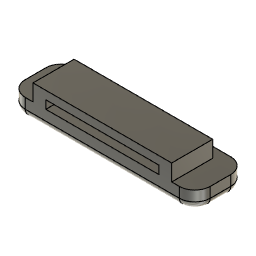
Keyboard_tray_end_stop_v5 (Autodesk Fusion 360 design; units mm, degrees)
Autodesk Fusion 360 part; units mm, degrees
sketch "Sketch1" plane through (0, 0, 0) normal (0, 0, 1) x (1, 0, 0)
  line L0 (0, 0) -> (36, 0)
  line L1 (36, 0) -> (36, 10)
  line L2 (36, 10) -> (0, 10)
  line L3 (0, 10) -> (0, 0)
  dimension "d1" = 10
  dimension "d2" = 36
  constraint horizontal L0
  constraint vertical L1
  constraint horizontal L2
  constraint vertical L3
  constraint coincident L0.start L3.end
  measures "d1" distance of L0 L2
  measures "d2" distance of L1 L3
extrude "Extrude1" add sketch "Sketch1" along normal blind 3.5
sketch "Sketch2" plane through (0, 0, 3.5) normal (0, 0, 1) x (-1, 0, 0)
  line L0 (0, -10) -> (0, 0)
  line L1 (0, 0) -> (-36, 0)
  line L2 (-36, 0) -> (-36, -10)
  line L3 (-36, -10) -> (0, -10)
  line L4 (-4.5, 0) -> (-31.5, 0)
  line L5 (-31.5, 0) -> (-31.5, -8)
  line L6 (-31.5, -8) -> (-4.5, -8)
  line L7 (-4.5, -8) -> (-4.5, 0)
  line L8 (0, -8) -> (-4.5, -8) construction
  line L9 (-31.5, -8) -> (-36, -8) construction
  dimension "d5" = 27
  dimension "d6" = 8
  constraint horizontal L4
  constraint vertical L5
  constraint horizontal L6
  constraint vertical L7
  constraint collinear L1 L4
  constraint coincident L0 L8.start
  constraint perpendicular L0 L8
  constraint coincident L2 L9.end
  constraint perpendicular L2 L9
  constraint equal L8 L9
  measures "d5" distance of L5 L7
  measures "d6" distance of L4 L6
extrude "Extrude2" add sketch "Sketch2" along normal blind 3.2 contours L1 L4 L5 L6 L7
sketch "Sketch3" plane through (0, 0, 0) normal (0, -1, 0) x (1, 0, 0)
  line L0 (0, 0) -> (36, 0)
  line L1 (36, 0) -> (36, 3.5)
  line L2 (36, 3.5) -> (31.5, 3.5)
  line L3 (31.5, 3.5) -> (31.5, 6.7)
  line L4 (31.5, 6.7) -> (4.5, 6.7)
  line L5 (4.5, 6.7) -> (4.5, 3.5)
  line L6 (4.5, 3.5) -> (0, 3.5)
  line L7 (0, 3.5) -> (0, 0)
  line L8 (4.5, 3.5) -> (31.5, 3.5) construction
  line L9 (7, 3.5) -> (29, 3.5)
  line L10 (29, 3.5) -> (29, 5.1)
  line L11 (29, 5.1) -> (7, 5.1)
  line L12 (7, 5.1) -> (7, 3.5)
  line L13 (7, 5.1) -> (4.5, 5.1) construction
  line L14 (29, 5.1) -> (31.5, 5.1) construction
  dimension "d9" = 22
  dimension "d10" = 1.6
  constraint coincident L5.end L6.start
  constraint coincident L2.end L3.start
  constraint horizontal L9
  constraint vertical L10
  constraint horizontal L11
  constraint vertical L12
  constraint coincident L8 L9.start
  constraint coincident L5 L13.end
  constraint perpendicular L5 L13
  constraint coincident L3 L14.end
  constraint perpendicular L3 L14
  constraint equal L13 L14
  measures "d9" distance of L10 L12
  measures "d10" distance of L8 L11
extrude "Extrude3" cut sketch "Sketch3" against normal through all contours L9 L10 L11 L12
fillet "Fillet1" radius 1.5 1 faces at (12, 6.6667, 0)
fillet "Fillet2" radius 3 8 edges at (35.5607, 0.4393, 0.4393) (36, 0, 2.5) (35.5607, 9.5607, 0.4393) (36, 10, 2.5) (0.4393, 0.4393, 0.4393) (0, 0, 2.5) (0.4393, 9.5607, 0.4393) (0, 10, 2.5)
equation "d1 = width"
equation "d2 = height"
equation "d3 = bumper_depth"
equation "d5 = runner_insert_height"
equation "d6 = width - runner_offset"
equation "d7 = runner_tab_thickness * 2"
equation "d9 = runner_tab_height"
equation "d10 = runner_tab_thickness"
equation "height = 36 mm"
equation "width = 10 mm"
equation "bumper_depth = 3.5 mm"
equation "runner_offset = 2 mm" comment "the amount the bumper overhangs the mounting block"
equation "runner_insert_height = 27 mm" comment "must be less than height"
equation "runner_tab_height = 22 mm" comment "must be less than runner_insert_height"
equation "runner_tab_thickness = 1.6 mm"
